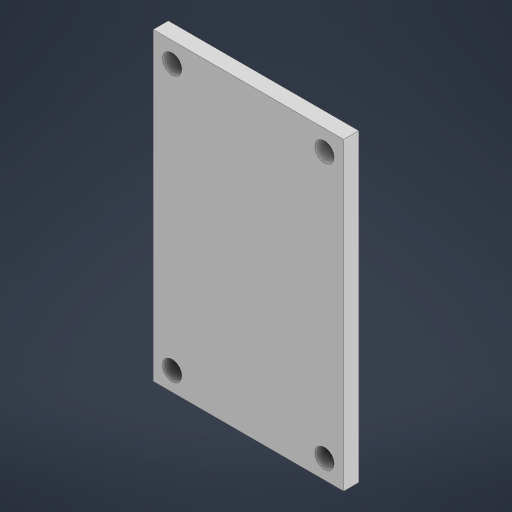
# Autodesk Inventor part: TurretMotorPlate
Saved by Autodesk Inventor 2024 (Build 280153000, 153)
## iProperties
Created: 2023-10-20
Part Number: TurretMotorPlate
Material: Generic
Document SubType Name: Modeling
Designer: avsar
Density: 1 g/cm^3
Appearance: Default
Author: avsar
Autodesk Inventor part; units mm, degrees
ref_plane "YZ Plane" through (0, 0, 0) normal (1, 0, 0) x (0, 1, 0)
ref_plane "XZ Plane" through (0, 0, 0) normal (0, 1, 0) x (-1, 0, 0)
ref_plane "XY Plane" through (0, 0, 0) normal (0, 0, 1) x (1, 0, 0)
sketch "Sketch1" plane through (0, 0, 0) normal (0, 0, 1) x (1, 0, 0)
  line L0 (-20, -32) -> (20, -32)
  line L1 (20, -32) -> (20, 32)
  line L2 (20, 32) -> (-20, 32)
  line L3 (-20, 32) -> (-20, -32)
  line L4 (-20, -32) -> (20, 32) construction
  line L5 (20, -32) -> (-20, 32) construction
  point P0 (0, 0)
  dimension "d0" = 40
  dimension "d1" = 64
  constraints: 12 end point, 2 midpoint, 2 parallel, 1 horizontal, 1 perpendicular
  measures "d0" distance of L2.end L1.end
  measures "d1" distance of L1.end L0.end
extrude "Extrusion1" add sketch "Sketch1" along normal blind 3.175
sketch "Sketch2" plane through (0, 0, 3.175) normal (0, 0, 1) x (1, 0, 0)
  circle A0 centre (-16, -28) radius 2
  line L0 (-20, -32) -> (20, -32) construction
  line L1 (20, -32) -> (20, 32) construction
  line L2 (20, 32) -> (-20, 32) construction
  line L3 (-20, 32) -> (-20, -32) construction
  line L4 (-20, -32) -> (20, -32) projected
  circle A1 centre (-16, 27.75) radius 2
  line L5 (0, 32) -> (0, -32) construction
  circle A2 centre (16, -28) radius 2
  circle A3 centre (16, 27.75) radius 2
  point P0 (0, 0)
  dimension "d4" = 4
  dimension "d5" = 4
  dimension "d6" = 16
  dimension "d7" = 4
  dimension "d8" = 59.75
  constraints: 4 centre point, 2 end point, 2 midpoint, 2 symmetric about line, 1 vertical alignment, 2 other
  measures "d4" diameter of A0
  measures "d5" distance from line of L0 A0.centre
  measures "d6" horizontal distance of point (0, 0) A0.centre
  measures "d7" diameter of A1
  measures "d8" distance from line of L0 A1.centre
extrude "Extrusion2" cut sketch "Sketch2" against normal through all
body "Solid1"
